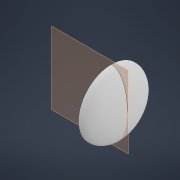
# Autodesk Inventor part: test spin toy
Saved by Autodesk Inventor 2022 (Build 260153000, 153)
## iProperties
Created: 2021-05-31
Part Number: test spin toy
Material: Generic
Document SubType Name: Modeling
Designer: sidsa
Density: 1 g/cm^3
Appearance: Default
Author: sidsa
## iProperties of the stored document test spin toy_3DPrint.ipt
Created: 2021-05-31
Part Number: test spin toy_3DPrint
Material: Generic
Document SubType Name: Modeling
Designer: sidsa
Density: 1 g/cm^3
Appearance: Default
Author: sidsa
Autodesk Inventor part; units mm, degrees
ref_plane "YZ Plane" through (0, 0, 0) normal (1, 0, 0) x (0, 1, 0)
ref_plane "XZ Plane" through (0, 0, 0) normal (0, 1, 0) x (-1, 0, 0)
sketch "Sketch1" plane through (0, 0, 0) normal (0, 0, 1) x (1, 0, 0)
  spline S0 degree 3 poles (0, 0) (5.236987, 6.284384) (10.473974, 12.584652) (15.71096, 17.928857) (19.454404, 21.748942) (23.197847, 25.090448) (26.941291, 27.408501) (29.661781, 29.09311) (32.382271, 30.245656) (35.10276, 30.449068) (37.023284, 30.592667) (38.943808, 30.272561) (40.864332, 29.131354) (42.169845, 28.355596) (43.475358, 27.211046) (44.780871, 25.372449) (45.631697, 24.174203) (46.482524, 22.693469) (47.333351, 20.622819) (47.862433, 19.335196) (48.391516, 17.83394) (48.920598, 15.820186) (49.229598, 14.644091) (49.538599, 13.309531) (49.847599, 11.528516) (50.002099, 10.638009) (50.156599, 9.644104) (50.311099, 8.355857) (50.38835, 7.711734) (50.4656, 6.998752) (50.54285, 6.09491) (50.581475, 5.642989) (50.6201, 5.145547) (50.658725, 4.530533) (50.679934, 4.192821) (50.701144, 3.821713) (50.722353, 3.364022) (50.738398, 3.017797) (50.754442, 2.640055) (50.770486, 2.076479) (50.771857, 2.028307) (50.773229, 1.978462) (50.7746, 1.92652) (50.783067, 1.605835) (50.791533, 1.204677) (50.8, 0) knots 0 0 0 0 0.30927087 0.30927087 0.30927087 0.53034038 0.53034038 0.53034038 0.69099922 0.69099922 0.69099922 0.80441598 0.80441598 0.80441598 0.8815132 0.8815132 0.8815132 0.93175888 0.93175888 0.93175888 0.9630039 0.9630039 0.9630039 0.98125195 0.98125195 0.98125195 0.99037597 0.99037597 0.99037597 0.99493799 0.99493799 0.99493799 0.99721899 0.99721899 0.99721899 0.99847153 0.99847153 0.99847153 0.99941901 0.99941901 0.99941901 0.9995 0.9995 0.9995 1 1 1 1
  line L0 (0, 0) -> (50.8, 0)
  constraints: 2 end point, 1 horizontal, 1 horizontal alignment, 2 other
revolve "Revolution1" add sketch "Sketch1" angle 360 about axis through (0, 0, 0) along (1, 0, 0)
sketch "Sketch2" plane through (0, 0, 0) normal (0, 0, 1) x (1, 0, 0)
  spline S0 degree 3 poles (50.8, 0) (50.791533, 1.204677) (50.783067, 1.605835) (50.7746, 1.92652) (50.773229, 1.978462) (50.771857, 2.028307) (50.770486, 2.076479) (50.754442, 2.640055) (50.738398, 3.017797) (50.722353, 3.364022) (50.701144, 3.821713) (50.679934, 4.192821) (50.658725, 4.530533) (50.6201, 5.145547) (50.581475, 5.642989) (50.54285, 6.09491) (50.4656, 6.998752) (50.38835, 7.711734) (50.311099, 8.355857) (50.156599, 9.644104) (50.002099, 10.638009) (49.847599, 11.528516) (49.538599, 13.309531) (49.229598, 14.644091) (48.920598, 15.820186) (48.391516, 17.83394) (47.862433, 19.335196) (47.333351, 20.622819) (46.482524, 22.693469) (45.631697, 24.174203) (44.780871, 25.372449) (43.475358, 27.211046) (42.169845, 28.355596) (40.864332, 29.131354) (38.943808, 30.272561) (37.023284, 30.592667) (35.10276, 30.449068) (32.382271, 30.245656) (29.661781, 29.09311) (26.941291, 27.408501) (23.197847, 25.090448) (19.454404, 21.748942) (15.71096, 17.928857) (10.473974, 12.584652) (5.236987, 6.284384) (0, 0) knots -2 -2 -2 -2 -1.999 -1.999 -1.999 -1.99883803 -1.99883803 -1.99883803 -1.99694305 -1.99694305 -1.99694305 -1.99443799 -1.99443799 -1.99443799 -1.98987597 -1.98987597 -1.98987597 -1.98075195 -1.98075195 -1.98075195 -1.9625039 -1.9625039 -1.9625039 -1.92600779 -1.92600779 -1.92600779 -1.86351776 -1.86351776 -1.86351776 -1.7630264 -1.7630264 -1.7630264 -1.60883195 -1.60883195 -1.60883195 -1.38199844 -1.38199844 -1.38199844 -1.06068075 -1.06068075 -1.06068075 -0.61854174 -0.61854174 -0.61854174 0 0 0 0
  line L0 (35.927173, 30.481181) -> (35.927173, -30.565071)
  line L1 (35.927173, -30.565071) -> (67.301693, -30.565071)
  line L2 (67.301693, -30.565071) -> (67.301693, 30.481181)
  line L3 (67.301693, 30.481181) -> (35.927173, 30.481181)
  line L4 (35.927173, 30.481181) -> (-48.061367, 30.481181)
  line L5 (-48.061367, 30.481181) -> (-48.061367, -59.26282)
  line L6 (-48.061367, -59.26282) -> (35.927173, -59.26282)
  line L7 (35.927173, -59.26282) -> (35.927173, 30.481181)
  point P0 (35.927173, -30.565071)
  constraints: 16 end point, 4 perpendicular, 2 parallel, 1 horizontal, 1 vertical, 3 other
extrude "Extrusion1" cut sketch "Sketch2" along normal mid plane 127 contours L0 L7 L6 L5 L4
body "Solid1"
